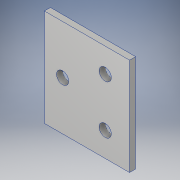
# Autodesk Inventor part: 2AM-17-P-0206 - moving support slider panl
Saved by Autodesk Inventor 2017 (Build 210142000, 142)
## iProperties
Created: 2017-12-27
Part Number: 2AM-17-P-0206 - moving support slider panl
Material: Aluminum 6061
Document SubType Name: Modeling
Designer: Micah
Density: 2.7 g/cm^3
Appearance: Aluminum - Flat
Mass: 169.821 g
Surface Area: 428.225 cm^2
Volume: 62.8966 cm^3
Author: Micah
Autodesk Inventor part; units mm, degrees
ref_plane "YZ Plane" through (0, 0, 0) normal (1, 0, 0) x (0, 1, 0)
ref_plane "XZ Plane" through (0, 0, 0) normal (0, 1, 0) x (-1, 0, 0)
ref_plane "XY Plane" through (0, 0, 0) normal (0, 0, 1) x (1, 0, 0)
sketch "Sketch1" plane through (0, 0, 0) normal (0, 0, 1) x (1, 0, 0)
  line L0 (355.6, 50.8) -> (-19.05, 50.8)
  line L1 (12.7, 50.8) -> (12.7, 0) construction
  line L2 (0, 38.1) -> (12.7, 38.1) construction
  line L3 (0, 12.7) -> (12.7, 12.7) construction
  circle A0 centre (12.7, 38.1) radius 3.175
  circle A1 centre (12.7, 12.7) radius 3.175
  line L4 (168.275, 50.8) -> (168.275, 0) construction
  line L5 (-19.05, 50.8) -> (-19.05, 0)
  line L6 (355.6, 50.8) -> (355.6, 0)
  circle A2 centre (-9.525, 25.4) radius 3.175
  circle A3 centre (323.85, 38.1) radius 3.175
  circle A4 centre (323.85, 12.7) radius 3.175
  line L7 (355.6, 50.8) -> (355.6, 0)
  circle A5 centre (346.075, 25.4) radius 3.175
  line L8 (-19.05, 0) -> (355.6, 0)
  dimension "d0" = 374.65
  dimension "d3" = 12.7
  dimension "d4" = 25.4
  dimension "d5" = 6.35
  dimension "d6" = 6.35
  dimension "d10" = 6.35
  dimension "d11" = 31.75
  constraints: 18 end point, 6 centre point, 5 point on line, 5 symmetric about line, 2 coincident, 2 perpendicular, 1 horizontal, 1 midpoint, 3 other
  measures "d0" distance of L0.end L0.start
  measures "d3" distance between parallel lines of L0 L2
  measures "d4" distance between parallel lines of L3 L2
  measures "d5" diameter of A0
  measures "d6" diameter of A1
  measures "d10" diameter of A2
  measures "d11" distance between parallel lines of L5 L1
extrude "Extrusion2" add sketch "Sketch1" along normal blind 3.175
sketch "Sketch3" plane through (0, 0, 3.175) normal (0, 0, 1) x (1, 0, 0)
  line L0 (-19.05, 50.8) -> (-19.05, 0) projected
  line L1 (-19.05, 25.4) -> (168.275, 25.4)
  line L2 (355.6, 50.8) -> (-19.05, 50.8) projected
  line L3 (168.275, 25.4) -> (168.275, 50.8)
  point P0 (0, 0)
  constraints: 4 end point, 2 midpoint, 1 parallel
hole "Hole1" at (168.275, 25.4, 3.175) direction (0, 0, -1) diameter 22.86 depth 25.4 tip angle 118
sketch "Sketch4" plane through (0, 0, 3.175) normal (0, 0, 1) x (1, 0, 0)
  circle A0 centre (168.275, 25.4) radius 11.43 projected
  line L0 (168.275, 25.4) -> (142.875, 25.4)
  circle A1 centre (142.875, 25.4) radius 3.175
  line L1 (355.6, 50.8) -> (-19.05, 50.8) projected
  line L2 (168.275, 50.8) -> (168.275, 0)
  circle A2 centre (193.675, 25.4) radius 3.175
  point P0 (0, 0)
  dimension "d21" = 25.4
  dimension "d22" = 6.35
  constraints: 4 end point, 2 centre point, 1 coincident, 1 horizontal, 1 midpoint, 1 symmetric about line, 1 vertical, 1 other
  measures "d21" distance of L0.start L0.end
  measures "d22" diameter of A1
hole "Hole2" at (193.675, 25.4, 3.175) at (142.875, 25.4, 3.175) direction (0, 0, -1) diameter 6.35 depth 25.4 tip angle 118
sketch "Sketch5" plane through (0, 0, 3.175) normal (0, 0, 1) x (1, 0, 0)
  line L0 (355.6, 50.8) -> (-19.05, 50.8) projected
  line L1 (74.6506, 50.8) -> (74.6506, 0)
  line L2 (-19.05, 50.8) -> (-19.05, 0) projected
  line L3 (74.6506, 50.8) -> (74.6506, 44.45)
  line L4 (74.6506, 44.45) -> (74.6506, 25.4)
  circle A0 centre (74.6506, 44.45) radius 2.0701
  line L5 (74.6506, 25.4) -> (74.6506, 6.35)
  circle A1 centre (74.6506, 25.4) radius 2.0701
  circle A2 centre (74.6506, 6.35) radius 2.0701
  line L6 (168.275, 50.8) -> (168.275, 0)
  circle A3 centre (261.8994, 44.45) radius 2.0701
  circle A4 centre (261.8994, 25.4) radius 2.0701
  circle A5 centre (261.8994, 6.35) radius 2.0701
  point P0 (0, 0)
  dimension "d30" = 93.7006
  dimension "d31" = 6.35
  dimension "d32" = 19.05
  dimension "d33" = 4.1402
  dimension "d34" = 19.05
  dimension "d35" = 4.1402
  dimension "d36" = 4.1402
  constraints: 10 end point, 6 centre point, 3 coincident, 3 point on line, 3 symmetric about line, 2 midpoint, 2 vertical, 3 other
  measures "d30" distance between parallel lines of L2 L1
  measures "d31" distance of L1.start L3.end
  measures "d32" distance of L3.end L4.end
  measures "d33" diameter of A0
  measures "d34" distance of L4.end L5.end
  measures "d35" diameter of A1
  measures "d36" diameter of A2
hole "Hole3" at (74.6506, 44.45, 3.175) at (74.6506, 25.4, 3.175) at (74.6506, 6.35, 3.175) at (261.8994, 44.45, 3.175) at (261.8994, 25.4, 3.175) at (261.8994, 6.35, 3.175) direction (0, 0, -1) diameter 4.1402 depth 25.4 tip angle 118
sketch "Sketch6" plane through (0, 0, 3.175) normal (0, 0, 1) x (1, 0, 0)
  circle A0 centre (12.7, 38.1) radius 3.175 projected
  line L0 (12.7, 38.1) -> (25.4, 38.1)
  line L1 (355.6, 50.8) -> (-19.05, 50.8) projected
  line L2 (25.4, 50.8) -> (25.4, 0)
  point P0 (0, 0)
  dimension "d44" = 12.7
  constraints: 4 end point, 1 horizontal, 1 point on line, 1 vertical
  measures "d44" distance of L0.start L0.end
split body "Split1" sketch "Sketch6" result one side removed curves L2 removed pieces at (41.1319, 25.4832, 0.5)
body "Solid2"
